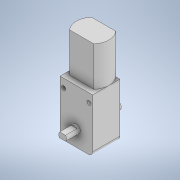
# Autodesk Inventor part: motor3
Saved by Autodesk Inventor 2020 (Build 240168000, 168)
## iProperties
Created: 2020-03-23
Part Number: motor3
Material: Generic
Document SubType Name: Modeling
Designer: Tarsoly
Density: 1 g/cm^3
Appearance: Default
Author: Tarsoly
Autodesk Inventor part; units mm, degrees
ref_plane "YZ Plane" through (0, 0, 0) normal (1, 0, 0) x (0, 1, 0)
ref_plane "XZ Plane" through (0, 0, 0) normal (0, 1, 0) x (-1, 0, 0)
ref_plane "XY Plane" through (0, 0, 0) normal (0, 0, 1) x (1, 0, 0)
sketch "Sketch1" plane through (0, 0, 0) normal (0, 1, 0) x (-1, 0, 0)
  line L0 (11.25, 9.4) -> (-11.25, 9.4)
  line L1 (-11.25, 9.4) -> (-11.25, -9.4)
  line L2 (-11.25, -9.4) -> (11.25, -9.4)
  line L3 (11.25, -9.4) -> (11.25, 9.4)
  line L4 (11.25, 9.4) -> (-11.25, -9.4) construction
  line L5 (-11.25, 9.4) -> (11.25, -9.4) construction
  point P0 (0, 0)
  dimension "d0" = 22.5
  dimension "d1" = 18.8
  constraints: 12 end point, 2 midpoint, 2 parallel, 1 horizontal, 1 perpendicular
  measures "d0" distance of L2.end L1.end
  measures "d1" distance of L1.end L0.end
extrude "Extrusion1" add sketch "Sketch1" along normal blind 37
sketch "Sketch2" plane through (-11.25, 0, 9.4) normal (0, 0, 1) x (1, 0, 0)
  circle A0 centre (11.25, 11.2) radius 2.7
  line L0 (0, 0) -> (22.5, 0) projected
  line L1 (11.25, 0) -> (11.25, 37) construction
  line L2 (0, 37) -> (22.5, 37) projected
  dimension "d4" = 5.4
  dimension "d5" = 11.2
  constraints: 2 end point, 1 centre point, 1 midpoint, 1 point on line, 1 vertical
  measures "d4" diameter of A0
  measures "d5" distance from line of L0 A0.centre
extrude "Extrusion2" add sketch "Sketch2" along normal blind 9.5
sketch "Sketch3" plane through (0, 11.2, 18.9) normal (0, 0, 1) x (1, 0, 0)
  circle A0 centre (0, 0) radius 2.7 projected
  line L0 (-2.0125, 1.8) -> (2.0125, 1.8)
  line L1 (-2.0125, -1.8) -> (2.0125, -1.8)
  point P0 (0, -11.2)
  dimension "d8" = 3.6
  constraints: 4 end point, 4 point on circle, 2 parallel, 1 horizontal
  measures "d8" distance between parallel lines of L1 L0
extrude "Extrusion3" cut sketch "Sketch3" against normal blind 7.9 contours L0 A0 | A0 L1
mirror "Mirror1" about plane through (0, 0, 0) normal (0, 0, 1) of "Extrusion2", "Extrusion3"
sketch "Sketch4" plane through (0, 0, 0) normal (0, -1, 0) x (1, 0, 0)
  line L0 (-2.5, -4.4) -> (2.5, -4.4)
  line L1 (2.5, -4.4) -> (2.5, -1.4)
  line L2 (2.5, -1.4) -> (-2.5, -1.4)
  line L3 (-2.5, -1.4) -> (-2.5, -4.4)
  line L4 (-2.5, -4.4) -> (2.5, -1.4) construction
  line L5 (2.5, -4.4) -> (-2.5, -1.4) construction
  line L6 (-11.25, 9.4) -> (11.25, 9.4) construction
  line L7 (0, -26.46) -> (0, 26.46) construction
  point P0 (0, -2.9)
  point P1 (0, -2.9)
  dimension "d11" = 5
  dimension "d12" = 3
  dimension "d22" = 10.8
  constraints: 12 end point, 3 midpoint, 2 parallel, 1 horizontal, 1 perpendicular, 1 point on line
  measures "d11" distance of L2.end L1.end
  measures "d12" distance of L1.end L0.end
  measures "d22" distance between parallel lines of L6 L2
extrude "Extrusion4" add sketch "Sketch4" along normal blind 5
sketch "Sketch5" plane through (2.5, 0, -4.4) normal (0, 0, -1) x (-1, 0, 0)
  circle A0 centre (2.5, -2.6) radius 1.4
  line L0 (5, -5) -> (0, -5) construction
  line L1 (2.5, 0) -> (2.5, -5) construction
  dimension "d15" = 2.8
  dimension "d16" = 2.4
  constraints: 2 end point, 1 centre point, 1 midpoint, 1 point on line
  measures "d15" diameter of A0
  measures "d16" distance from line of L0 A0.centre
extrude "Extrusion5" cut sketch "Sketch5" against normal up to next
sketch "Sketch6" plane through (0, 37, 0) normal (0, 1, 0) x (1, 0, 0)
  line L0 (11.25, 9.4) -> (-11.25, 9.4) projected
  line L1 (11.25, -9.4) -> (11.25, 9.4) projected
  line L2 (-11.25, 9.4) -> (11.25, 9.4)
  line L3 (11.25, 9.4) -> (11.25, -5.7)
  line L4 (11.25, -5.7) -> (-11.25, -5.7)
  line L5 (-11.25, -5.7) -> (-11.25, 9.4)
  line L6 (-11.25, -9.4) -> (11.25, -9.4) projected
  circle A0 centre (0, 1.85) radius 11.25
  line L7 (-11.25, 9.4) -> (-11.25, -9.4) projected
  line L8 (11.25, -9.4) -> (11.25, 9.4) projected
  point P0 (0, 0)
  point P1 (-8.3403, 9.4)
  point P2 (-8.3403, -5.7)
  point P3 (8.3403, -5.7)
  point P4 (8.3403, 9.4)
  dimension "d19" = 3.7
  dimension "d23" = 15.1
  dimension "d24" = 7.55
  constraints: 8 end point, 2 parallel, 2 tangent, 1 centre point, 1 horizontal, 1 perpendicular, 1 point on line
  measures "d19" distance between parallel lines of L4 L6
  measures "d23" distance between parallel lines of L4 L0
  measures "d24" distance from line of L0 A0.centre
extrude "Extrusion6" add sketch "Sketch6" along normal blind 27.2 contours A0 L4 L0
sketch "Sketch7" plane through (-11.25, 0, 9.4) normal (0, 0, 1) x (1, 0, 0)
  circle A0 centre (2.5, 31.1) radius 1.4
  line L0 (0, 0) -> (22.5, 0) projected
  line L1 (0, 37) -> (22.5, 37) construction
  circle A1 centre (20, 31.1) radius 1.4
  line L2 (0, 0) -> (0, 37) projected
  point P0 (11.25, 0)
  dimension "d25" = 2.8
  dimension "d26" = 31.1
  dimension "d29" = 17.5
  dimension "d34" = 22.5
  dimension "d35" = 2.5
  constraints: 2 centre point, 1 horizontal, 2 other
  measures "d25" diameter of A0
  measures "d26" distance from line of L0 A0.centre
  measures "d29" distance of A0.centre A1.centre
  measures "d34" distance of L1.start L1.end
  measures "d35" distance from line of L2 A0.centre
extrude "Extrusion7" cut sketch "Sketch7" against normal blind 4
fillet "Fillet1" radius 3 2 edges at (11.25, 0, 0) (-11.25, 0, 0)
equation "\"d24\" = 0.5 * d23"
equation "\"d35\" = -0.5 * d29 + 0.5 * d34"
body "Solid1"
